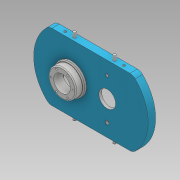
# Autodesk Inventor part: 밑판(new)
Saved by Autodesk Inventor 2018 (Build 220112000, 112)
## iProperties
Created: 2018-04-19
Part Number: 밑판(new)
Material: 일반
Document SubType Name: Modeling
Designer: CK
Density: 1 g/cm^3
Appearance: 기본값
Author: CK
Autodesk Inventor part; units mm, degrees
ref_plane "YZ Plane" through (0, 0, 0) normal (1, 0, 0) x (0, 1, 0)
ref_plane "XZ Plane" through (0, 0, 0) normal (0, 1, 0) x (-1, 0, 0)
ref_plane "XY Plane" through (0, 0, 0) normal (0, 0, 1) x (1, 0, 0)
sketch "스케치1" plane through (0, 0, 0) normal (0, 1, 0) x (-1, 0, 0)
  line L0 (-45, 36) -> (45, 36)
  line L1 (45, 36) -> (45, -36)
  line L2 (45, -36) -> (-45, -36)
  line L3 (-45, -36) -> (-45, 36)
  line L4 (-45, 36) -> (45, -36) construction
  line L5 (45, 36) -> (-45, -36) construction
  arc A0 (45, -36) -> (45, 36) centre (14.036557, 0) ccw
  line L6 (0, 68.394067) -> (0, -86.625) construction
  arc A1 (-45, 36) -> (-45, -36) centre (-14.036557, 0) ccw
  point P0 (0, 0)
  dimension "d0" = 90
  dimension "d1" = 72
  constraints: 14 end point, 4 point on circle, 2 centre point, 2 midpoint, 2 parallel, 1 horizontal, 1 perpendicular, 1 symmetric about line, 1 vertical, 1 other
  measures "d0" distance of L1.end L2.end
  measures "d1" distance of L0.end L1.end
sketch "스케치1 outline for 돌출1" plane through (0, 0, 0) normal (0, 1, 0) x (-1, 0, 0)
  arc A0 (-45, 36) -> (-45, -36) centre (-14.036557, 0) ccw
  line L0 (-45, -36) -> (45, -36)
  arc A1 (45, -36) -> (45, 36) centre (14.036557, 0) ccw
  line L1 (45, 36) -> (-45, 36)
extrude "돌출1" add sketch "스케치1 outline for 돌출1" along normal blind 8
fillet "모깎기1" radius 8 4 edges at (45, 4, 36) (-45, 4, 36) (-45, 4, -36) (45, 4, -36)
shell "쉘1" thickness 5 removed faces 1 at (-13.9584, 8, 12)
sketch "스케치2" plane through (0, 0, 0) normal (0, -1, 0) x (1, 0, 0)
  circle A0 centre (-21, 0) radius 15
  circle A1 centre (-21, 0) radius 16.25
  point P0 (0, 0)
  dimension "d6" = 21
  dimension "d7" = 30
  dimension "d8" = 32.5
  constraints: 2 centre point, 1 coincident
  measures "d6" distance of A0.centre point (0, 0)
  measures "d7" diameter of A0
  measures "d8" diameter of A1
sketch "스케치2 outline for 돌출2" plane through (0, 0, 0) normal (0, -1, 0) x (1, 0, 0)
  circle A0 centre (-21, 0) radius 16.25
extrude "돌출2" add sketch "스케치2 outline for 돌출2" along normal blind 3
sketch "스케치3" plane through (-21, -3, 0) normal (0, -1, 0) x (1, 0, 0)
  circle A0 centre (0, 0) radius 14.75
  point P0 (21, 0)
  dimension "d11" = 29.5
  constraints: 1 centre point
  measures "d11" diameter of A0
sketch "스케치3 outline for 돌출3" plane through (-21, -3, 0) normal (0, -1, 0) x (1, 0, 0)
  circle A0 centre (0, 0) radius 14.75
extrude "돌출3" add sketch "스케치3 outline for 돌출3" along normal blind 7
sketch "스케치4" plane through (-21, -10, 0) normal (0, -1, 0) x (1, 0, 0)
  circle A0 centre (0, 0) radius 9
  point P0 (21, 0)
  dimension "d14" = 18
  constraints: 1 centre point
  measures "d14" diameter of A0
sketch "스케치4 outline for 돌출4" plane through (-21, -10, 0) normal (0, -1, 0) x (1, 0, 0)
  circle A0 centre (0, 0) radius 9
extrude "돌출4" cut sketch "스케치4 outline for 돌출4" against normal through all
fillet "모깎기2" radius 1 1 edges at (-35.75, -10, 0)
sketch "스케치5" plane through (0, 0, 0) normal (0, -1, 0) x (1, 0, 0)
  circle A0 centre (-21, 0) radius 9 projected
  circle A1 centre (17.5, 0) radius 9
  point P0 (0, 0)
  dimension "d18" = 18
  dimension "d19" = 38.5
  constraints: 1 centre point
  measures "d18" diameter of A1
  measures "d19" distance of A0.centre A1.centre
sketch "스케치5 outline for 돌출5" plane through (0, 0, 0) normal (0, -1, 0) x (1, 0, 0)
  circle A0 centre (17.5, 0) radius 9
extrude "돌출5" cut sketch "스케치5 outline for 돌출5" against normal blind 10
sketch "스케치6" plane through (-21, -10, 0) normal (0, -1, 0) x (1, 0, 0)
  circle A0 centre (0, 0) radius 12 construction
  circle A1 centre (-12, 0) radius 0.9
  point P0 (21, 0)
  dimension "d22" = 24
  dimension "d23" = 1.8
  constraints: 1 centre point, 1 horizontal alignment, 2 other
  measures "d23" diameter of A1
sketch "스케치6 outline for 돌출6" plane through (-21, -10, 0) normal (0, -1, 0) x (1, 0, 0)
  circle A0 centre (-12, 0) radius 0.9
extrude "돌출6" cut sketch "스케치6 outline for 돌출6" against normal blind 5
pattern_circular "원형 패턴1" count 6 over 360 about axis through (-21, -10, 0) along (0, 1, 0) of "돌출6"
sketch "스케치7" plane through (0, 0, 0) normal (0, -1, 0) x (1, 0, 0)
  circle A0 centre (17.5, 0) radius 9 projected
  circle A1 centre (17.5, 21.915) radius 1.5
  circle A2 centre (17.5, -21.915) radius 2
  point P0 (0, 0)
  dimension "d29" = 3
  dimension "d30" = 21.915
  dimension "d31" = 4
  dimension "d32" = 21.915
  constraints: 2 centre point
  measures "d29" diameter of A1
  measures "d30" distance of A0.centre A1.centre
  measures "d31" diameter of A2
  measures "d32" distance of A2.centre A0.centre
sketch "스케치7 outline for 돌출7" plane through (0, 0, 0) normal (0, -1, 0) x (1, 0, 0)
  circle A0 centre (17.5, 21.915) radius 1.5
  circle A1 centre (17.5, -21.915) radius 2
extrude "돌출7" cut sketch "스케치7 outline for 돌출7" against normal blind 7
sketch "스케치9" plane through (-41.8752, 0, 36) normal (0, 0, 1) x (1, 0, 0)
  line L0 (-3.355128, 4) -> (110.237879, 4) construction
  line L1 (0, 0) -> (83.7504, 0)
  line L2 (20.3752, 11.284073) -> (20.3752, -22.756214) construction
  line L3 (10.3752, 14.199125) -> (10.3752, -23.790588) construction
  line L4 (41.8752, 0) -> (41.8752, 28.304217) construction
  line L5 (63.3752, 11.284073) -> (63.3752, -22.756214) construction
  line L6 (73.3752, 14.199125) -> (73.3752, -23.790588) construction
  circle A0 centre (20.3752, 4) radius 1.5
  circle A1 centre (63.3752, 4) radius 1.5
  dimension "d39" = 4
  dimension "d40" = 31.5
  dimension "d41" = 21.5
  dimension "d42" = 3
  dimension "d43" = 3
  constraints: 12 end point, 4 point on line, 4 symmetric about line, 3 vertical, 2 centre point, 1 horizontal
  measures "d39" distance between parallel lines of L1 L0
  measures "d40" distance from line of L4.start L3
  measures "d41" distance from line of L4.start L2
  measures "d42" diameter of A0
  measures "d43" diameter of A1
sketch "스케치9 outline for 돌출9" plane through (-41.8752, 0, 36) normal (0, 0, 1) x (1, 0, 0)
  circle A0 centre (20.3752, 4) radius 1.5
  circle A1 centre (63.3752, 4) radius 1.5
extrude "돌출9" add sketch "스케치9 outline for 돌출9" along normal blind 5
sketch "스케치10" plane through (-41.8752, 0, 36) normal (0, 0, 1) x (1, 0, 0)
  line L0 (-42.215382, 4) -> (125.010207, 4) construction
  line L1 (10.3752, 32.808069) -> (10.3752, -49.68989)
  line L2 (73.3752, 21.181908) -> (73.3752, -27.233882)
  circle A0 centre (10.3752, 4) radius 1.25
  circle A1 centre (73.3752, 4) radius 1.25
  point P0 (41.8752, 0)
  dimension "d46" = 4
  dimension "d47" = 31.5
  dimension "d48" = 31.5
  dimension "d49" = 2.5
  dimension "d50" = 2.5
  constraints: 6 end point, 4 point on line, 2 centre point, 2 vertical, 1 horizontal
  measures "d46" distance from line of point (41.875, 0) L0
  measures "d47" distance from line of point (41.875, 0) L1
  measures "d48" distance from line of L2 point (41.875, 0)
  measures "d49" diameter of A0
  measures "d50" diameter of A1
sketch "스케치10 outline for 돌출10" plane through (-41.8752, 0, 36) normal (0, 0, 1) x (1, 0, 0)
  circle A0 centre (10.3752, 4) radius 1.25
  circle A1 centre (73.3752, 4) radius 1.25
extrude "돌출10" cut sketch "스케치10 outline for 돌출10" against normal blind 8.8
fillet "모깎기3" radius 1 1 edges at (-37.25, -3, 0)
mirror "미러2" about plane through (0, 0, 0) normal (0, 0, 1) of "돌출10", "돌출9"
sketch "스케치12" plane through (-14.036557, 5, 0) normal (0, 1, 0) x (1, 0, 0)
  arc A0 (-29.953824, 30.127441) -> (-29.953824, -30.127441) centre (0, 0) ccw
  arc A1 (-27.838642, 31) -> (-29.953824, 30.127441) centre (-27.838642, 28) ccw
  line L0 (-27.838642, 31) -> (55.911757, 31)
  arc A2 (58.026939, 30.127441) -> (55.911757, 31) centre (55.911757, 28) ccw
  arc A3 (58.026939, -30.127441) -> (58.026939, 30.127441) centre (28.073115, 0) ccw
  arc A4 (55.911757, -31) -> (58.026939, -30.127441) centre (55.911757, -28) ccw
  line L1 (55.911757, -31) -> (-27.838642, -31)
  arc A5 (-29.953824, -30.127441) -> (-27.838642, -31) centre (-27.838642, -28) ccw
  point P0 (14.036557, 0)
sketch "스케치12 outline for 돌출12" plane through (-14.036557, 5, 0) normal (0, 1, 0) x (1, 0, 0)
  arc A0 (-29.953824, -30.127441) -> (-29.953824, 30.127441) centre (0, 0) cw
  arc A1 (-29.953824, 30.127441) -> (-27.838642, 31) centre (-27.838642, 28) cw
  line L0 (-27.838642, 31) -> (55.911757, 31)
  arc A2 (55.911757, 31) -> (58.026939, 30.127441) centre (55.911757, 28) cw
  arc A3 (58.026939, 30.127441) -> (58.026939, -30.127441) centre (28.073115, 0) cw
  arc A4 (58.026939, -30.127441) -> (55.911757, -31) centre (55.911757, -28) cw
  line L1 (55.911757, -31) -> (-27.838642, -31)
  arc A5 (-27.838642, -31) -> (-29.953824, -30.127441) centre (-27.838642, -28) cw
extrude "돌출12" cut sketch "스케치12 outline for 돌출12" against normal blind 2
sketch "스케치13" plane through (41.8752, 8, 31) normal (0, 0, -1) x (-1, 0, 0)
  arc A0 (74.1252, -5) -> (72.6252, -5) centre (73.3752, -4) ccw projected
  circle A1 centre (73.3752, -4) radius 1.25
  circle A2 centre (73.3752, -4) radius 1.75
  point P0 (41.8752, -8)
  dimension "d59" = 3.5
  constraints: 2 centre point, 2 coincident, 1 concentric
  measures "d59" diameter of A2
sketch "스케치13 outline for 돌출13" plane through (41.8752, 8, 31) normal (0, 0, -1) x (-1, 0, 0)
  circle A0 centre (73.3752, -4) radius 1.75
  circle A1 centre (73.3752, -4) radius 1.25
extrude "돌출13" add sketch "스케치13 outline for 돌출13" along normal blind 4
mirror "미러3" about plane through (0, 0, 0) normal (1, 0, 0) of "돌출13"
mirror "미러4" about plane through (0, 0, 0) normal (0, 0, 1) of "돌출13", "미러3"
sketch "스케치14" plane through (-14.036557, 3, 0) normal (0, 1, 0) x (1, 0, 0)
  arc A0 (-17.963443, -8.660254) -> (-17.963443, 8.660254) centre (-6.963443, 0) ccw
  line L0 (-17.963443, -8.660254) -> (-17.963443, 8.660254)
  point P0 (14.036557, 0)
  dimension "d62" = 28
  dimension "d63" = 25
  constraints: 2 end point, 2 point on circle, 1 centre point, 1 coincident, 1 vertical
  measures "d62" diameter of A0
sketch "스케치14 outline for 돌출14" plane through (-14.036557, 3, 0) normal (0, 1, 0) x (1, 0, 0)
  line L0 (-17.963443, 8.660254) -> (-17.963443, -8.660254)
  arc A0 (-17.963443, -8.660254) -> (-17.963443, 8.660254) centre (-6.963443, 0) ccw
extrude "돌출14" cut sketch "스케치14 outline for 돌출14" against normal blind 3
sketch "스케치15" plane through (-14.036557, 0, 0) normal (0, 1, 0) x (1, 0, 0)
  circle A0 centre (-6.963443, 0) radius 12.75 construction
  circle A1 centre (5.786557, 0) radius 0.9
  circle A2 centre (-13.338443, 11.041824) radius 0.9
  circle A3 centre (-13.338443, -11.041824) radius 0.9
  point P0 (14.036557, 0)
  dimension "d66" = 25.5
  dimension "d67" = 1.8
  dimension "d70" = 360
  constraints: 3 centre point, 1 coincident, 1 horizontal alignment, 9 other
  measures "d67" diameter of A1
sketch "스케치15 outline for 돌출15" plane through (-14.036557, 0, 0) normal (0, 1, 0) x (1, 0, 0)
  circle A0 centre (5.786557, 0) radius 0.9
  circle A1 centre (-13.338443, 11.041824) radius 0.9
  circle A2 centre (-13.338443, -11.041824) radius 0.9
extrude "돌출15" cut sketch "스케치15 outline for 돌출15" against normal blind 3
